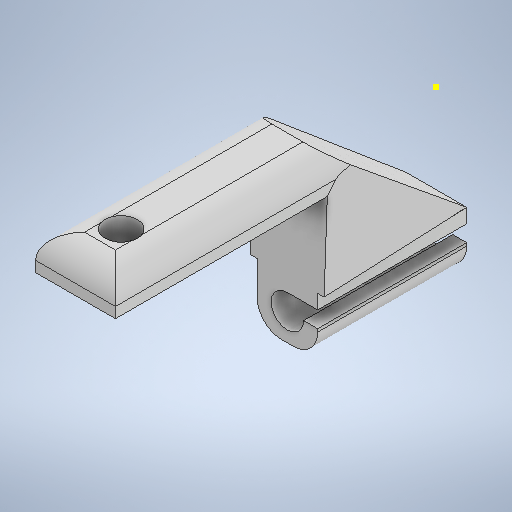
# Autodesk Inventor part: Part3
Saved by Autodesk Inventor 2025.3 (Build 293356000, 356)
## iProperties
Created: 2025-07-14
Part Number: Part3
Material: Generic
Document SubType Name: Modeling
Designer: steve
Density: 1 g/cm^3
Appearance: Default
Author: steve
Autodesk Inventor part; units mm, degrees
ref_plane "YZ Plane" through (0, 0, 0) normal (1, 0, 0) x (0, 1, 0)
ref_plane "XZ Plane" through (0, 0, 0) normal (0, 1, 0) x (-1, 0, 0)
ref_plane "XY Plane" through (0, 0, 0) normal (0, 0, 1) x (1, 0, 0)
sketch "Sketch1" plane through (0, 0, 0) normal (0, 1, 0) x (-1, 0, 0)
  circle A0 centre (0, 0) radius 1
  line L0 (0, 1) -> (0, 2.8)
  line L1 (-2.45, 2.8) -> (2.45, 2.8)
  line L2 (2.45, 2.8) -> (2.45, -10.2)
  line L3 (2.45, -10.2) -> (-2.45, -10.2)
  line L4 (-2.45, -10.2) -> (-2.45, 2.8)
  dimension "d0" = 2
  dimension "d1" = 1.8
  dimension "d2" = 4.9
  dimension "d3" = 13
  constraints: 10 end point, 2 perpendicular, 2 vertical, 1 coincident, 1 horizontal, 1 midpoint, 1 vertical alignment, 2 other
  measures "d1" distance of L0.end L0.start
  measures "d2" distance of L1.start L1.end
  measures "d3" distance of L1.end L2.end
extrude "Extrusion1" add sketch "Sketch1" along normal blind 2.15
sketch "Sketch2" plane through (2.45, 0, 2.8) normal (1, 0, 0) x (0, 0, -1)
  line L0 (0, 0) -> (13, 0) projected
  line L1 (13, 2.15) -> (13, -5.45)
  line L2 (13, -5.45) -> (22.15, -5.45)
  line L3 (13, 2.15) -> (22.15, -5.45)
  point P0 (2.8, 0)
  dimension "d6" = 7.6
  dimension "d7" = 9.15
  constraints: 6 end point, 1 coincident, 1 perpendicular, 1 vertical
  measures "d6" distance of L1.start L1.end
  measures "d7" distance of L1.end L2.end
extrude "Extrusion2" add sketch "Sketch2" against normal up to surface (4.9 mm away)
sketch "Sketch3" plane through (-2.45, 2.15, -10.2) normal (0, 0.7692539, -0.6389432) x (1, 0, 0)
  line L0 (4.31, 11.8946) -> (0.59, 11.8946)
  line L1 (4.9, 11.8946) -> (0, 11.8946) projected
  line L2 (4.9, -8.6266) -> (4.9, 1.3737) projected
  line L3 (4.31, 11.8946) -> (4.9, 1.3737)
  line L4 (0, 1.3737) -> (0, -8.6266) projected
  line L5 (0.59, 11.8946) -> (0, 1.3737)
  line L6 (4.9, 1.3737) -> (0, 1.3737) projected
  line L7 (4.9, 1.3737) -> (4.9, 11.8946)
  line L8 (4.9, 11.8946) -> (4.31, 11.8946)
  line L9 (0.59, 11.8946) -> (0, 11.8946)
  line L10 (0, 11.8946) -> (0, 1.3737)
  point P0 (2.45, -6.4727)
  point P1 (2.45, 11.8946)
  point P2 (0.59, 11.8946)
  point P3 (4.31, 11.8946)
  dimension "d10" = 3.72
  constraints: 14 end point, 3 perpendicular, 2 midpoint, 1 collinear, 1 horizontal
  measures "d10" distance of L0.start L0.end
extrude "Extrusion3" cut sketch "Sketch3" against normal blind 10 contours L1 L7 L3 | L5 L10 L1
sketch "Sketch4" plane through (-2.2547, -5.45, -10.2) normal (0, -1, 0) x (1, 0, 0)
  line L0 (4.1147, -9.15) -> (0.3947, -9.15) projected
  line L1 (4.7047, 0) -> (-0.1953, 0) projected
  line L2 (4.1147, -9.15) -> (0.3947, -9.15)
  line L3 (0.3947, -9.15) -> (0.3947, 0)
  line L4 (0.3947, 0) -> (4.1147, 0)
  line L5 (4.1147, 0) -> (4.1147, -9.15)
  point P0 (2.2547, 10.2)
  dimension "d13" = 3.72
  constraints: 8 end point, 2 parallel, 1 horizontal, 1 perpendicular, 1 point on line
  measures "d13" distance between parallel lines of L5 L3
extrude "Extrusion4" add sketch "Sketch4" along normal blind 3.56
fillet "Fillet1" radius 1.5 2 edges at (1.86, -9.01, -14.775) (-1.86, -9.01, -14.775)
sketch "Sketch5" plane through (1.86, -5.45, -19.35) normal (0, 0, -1) x (-1, 0, 0)
  circle A0 centre (1.86, -1.875) radius 1
  line L0 (1.86, -0.875) -> (-0.4108, -0.875)
  line L1 (-0.4108, -0.875) -> (-0.4108, -1.875)
  line L2 (-0.4108, -1.875) -> (0.86, -1.875)
  point P0 (1.86, 5.45)
  dimension "d17" = 2
  constraints: 6 end point, 2 perpendicular, 2 point on circle, 1 centre point, 1 horizontal, 1 tangent
  measures "d17" diameter of A0
extrude "Extrusion5" cut sketch "Sketch5" against normal through all contours A0
sketch "Sketch6" plane through (1.86, -5.45, -19.35) normal (0, 0, -1) x (-1, 0, 0)
  point P0 (1.86, 5.45)
extrude "Extrusion6" cut sketch "Sketch5" against normal through all contours A0 L2 L1 L0
fillet "Fillet2" radius 1.5 3 edges at (2.45, 2.15, -3.7) (-2.45, 2.15, -3.7) (0, 2.15, 2.8)
body "Solid1"
